Autodesk Fusion 360 part; units mm, degrees
note: some values were not read from the file. Chosen so that the rebuilt part matches the saved one: which bodies a step acts on; which sketch regions a step uses.
(part 3 of 6)
  line L723 (-60.9101, -10.8648) -> (-58.4101, -10.8648)
  line L724 (-6.5, -11.4513) -> (-5.25, -13.6164)
  line L725 (-55.8611, -13.6164) -> (-53.3611, -13.6164)
  line L726 (-68.5324, -10.8648) -> (-67.2824, -8.6997)
  line L727 (-76.1056, -7.9497) -> (-73.6056, -7.9497)
  line L728 (-92.5268, -8.6997) -> (-91.2768, -10.8648)
  line L729 (-72.2824, -8.6997) -> (-71.0324, -10.8648)
  line L730 (-10.299, -12.2013) -> (-11.549, -14.3664)
  line L731 (-5.25, -9.2863) -> (-6.5, -11.4513)
  line L732 (-101.399, -6.5347) -> (-102.649, -8.6997)
  line L733 (-65.9833, -3.6196) -> (-67.2333, -5.7847)
  line L734 (-63.4833, -7.9497) -> (-62.2333, -5.7847)
  line L735 (-71.0324, -10.8648) -> (-68.5324, -10.8648)
  line L736 (-81.1546, -6.5347) -> (-82.4046, -8.6997)
  line L737 (-7.799, -12.2013) -> (-10.299, -12.2013)
  line L738 (-58.4101, -6.5347) -> (-60.9101, -6.5347)
  line L739 (-83.7278, -3.6196) -> (-86.2278, -3.6196)
  line L740 (-2.75, -9.2863) -> (-5.25, -9.2863)
  line L741 (-77.4046, -8.6997) -> (-78.6546, -6.5347)
  line L742 (-10.299, -16.5315) -> (-7.799, -16.5315)
  line L743 (-11.549, -14.3664) -> (-10.299, -16.5315)
  line L744 (-60.9101, -6.5347) -> (-62.1601, -8.6997)
  line L745 (-86.2278, -3.6196) -> (-87.4778, -5.7847)
  line L746 (-15.3722, -13.6164) -> (-12.8722, -13.6164)
  line L747 (-22.9944, -9.2863) -> (-25.4944, -9.2863)
  line L748 (-26.7935, -14.3664) -> (-28.0435, -12.2013)
  line L749 (-48.2879, -12.2013) -> (-50.7879, -12.2013)
  line L750 (-53.3611, -9.2863) -> (-55.8611, -9.2863)
  line L751 (-15.3722, -9.2863) -> (-16.6222, -11.4513)
  line L752 (-46.9889, -11.4513) -> (-45.7389, -13.6164)
  line L753 (-35.6167, -13.6164) -> (-33.1167, -13.6164)
  line L754 (-31.7935, -14.3664) -> (-30.5435, -16.5315)
  line L755 (-6.549, -14.3664) -> (-7.799, -12.2013)
  line L756 (-17.9213, -12.2013) -> (-20.4213, -12.2013)
  line L757 (-60.9101, -12.2013) -> (-62.1601, -14.3664)
  line L758 (-40.6657, -12.2013) -> (-41.9157, -14.3664)
  line L759 (-53.3611, -13.6164) -> (-52.1111, -11.4513)
  line L760 (-26.7444, -11.4513) -> (-25.4944, -13.6164)
  line L761 (-41.9157, -14.3664) -> (-40.6657, -16.5315)
  line L762 (-50.7879, -16.5315) -> (-48.2879, -16.5315)
  line L763 (-60.9101, -16.5315) -> (-58.4101, -16.5315)
  line L764 (-58.4101, -12.2013) -> (-60.9101, -12.2013)
  line L765 (-67.2333, -11.4513) -> (-65.9833, -13.6164)
  line L766 (-28.0435, -16.5315) -> (-26.7935, -14.3664)
  line L767 (-17.9213, -16.5315) -> (-16.6713, -14.3664)
  line L768 (-47.0379, -14.3664) -> (-48.2879, -12.2013)
  line L769 (-12.8722, -13.6164) -> (-11.6222, -11.4513)
  line L770 (-35.6167, -9.2863) -> (-36.8667, -11.4513)
  line L771 (-43.2389, -9.2863) -> (-45.7389, -9.2863)
  line L772 (-57.1111, -11.4513) -> (-55.8611, -13.6164)
  line L773 (-33.1167, -9.2863) -> (-35.6167, -9.2863)
  line L774 (-48.2879, -16.5315) -> (-47.0379, -14.3664)
  line L775 (-30.5435, -16.5315) -> (-28.0435, -16.5315)
  line L776 (-45.7389, -13.6164) -> (-43.2389, -13.6164)
  line L777 (-58.4101, -16.5315) -> (-57.1601, -14.3664)
  line L778 (-30.5435, -12.2013) -> (-31.7935, -14.3664)
  line L779 (-52.0379, -14.3664) -> (-50.7879, -16.5315)
  line L780 (-45.7389, -9.2863) -> (-46.9889, -11.4513)
  line L781 (-55.8611, -9.2863) -> (-57.1111, -11.4513)
  line L782 (-36.9157, -14.3664) -> (-38.1657, -12.2013)
  line L783 (-50.7879, -12.2013) -> (-52.0379, -14.3664)
  line L784 (-43.2389, -13.6164) -> (-41.9889, -11.4513)
  line L785 (-36.8667, -11.4513) -> (-35.6167, -13.6164)
  line L786 (-22.9944, -13.6164) -> (-21.7444, -11.4513)
  line L787 (-20.4213, -16.5315) -> (-17.9213, -16.5315)
  line L788 (-21.6713, -14.3664) -> (-20.4213, -16.5315)
  line L789 (-52.1111, -11.4513) -> (-53.3611, -9.2863)
  line L790 (-28.0435, -12.2013) -> (-30.5435, -12.2013)
  line L791 (-20.4213, -12.2013) -> (-21.6713, -14.3664)
  line L792 (-25.4944, -9.2863) -> (-26.7444, -11.4513)
  line L793 (-7.799, -16.5315) -> (-6.549, -14.3664)
  line L794 (-57.1601, -14.3664) -> (-58.4101, -12.2013)
  line L795 (-12.8722, -9.2863) -> (-15.3722, -9.2863)
  line L796 (-65.9833, -13.6164) -> (-63.4833, -13.6164)
  line L797 (-25.4944, -13.6164) -> (-22.9944, -13.6164)
  line L798 (-40.6657, -16.5315) -> (-38.1657, -16.5315)
  line L799 (-31.8667, -11.4513) -> (-33.1167, -9.2863)
  line L800 (-41.9889, -11.4513) -> (-43.2389, -9.2863)
  line L801 (-38.1657, -12.2013) -> (-40.6657, -12.2013)
  line L802 (-62.1601, -14.3664) -> (-60.9101, -16.5315)
  line L803 (-11.6222, -11.4513) -> (-12.8722, -9.2863)
  line L804 (-21.7444, -11.4513) -> (-22.9944, -9.2863)
  line L805 (-16.6222, -11.4513) -> (-15.3722, -13.6164)
  line L806 (-68.5324, -16.5315) -> (-67.2824, -14.3664)
  line L807 (-38.1657, -16.5315) -> (-36.9157, -14.3664)
  line L808 (-67.2824, -14.3664) -> (-68.5324, -12.2013)
  line L809 (-62.1601, -76.6997) -> (-60.9101, -78.8648)
  line L810 (-86.2278, -71.6196) -> (-87.4778, -73.7847)
  line L811 (-97.6, -73.7847) -> (-96.35, -75.9497)
  line L812 (-87.4778, -73.7847) -> (-86.2278, -75.9497)
  line L813 (-76.1056, -75.9497) -> (-73.6056, -75.9497)
  line L814 (-78.6546, -78.8648) -> (-77.4046, -76.6997)
  line L815 (-77.4046, -76.6997) -> (-78.6546, -74.5347)
  line L816 (-71.0324, -78.8648) -> (-68.5324, -78.8648)
  line L817 (-63.4833, -13.6164) -> (-62.2333, -11.4513)
  line L818 (-33.1167, -13.6164) -> (-31.8667, -11.4513)
  line L819 (-63.4833, -9.2863) -> (-65.9833, -9.2863)
  line L820 (-72.2824, -14.3664) -> (-71.0324, -16.5315)
  line L821 (-71.0324, -12.2013) -> (-72.2824, -14.3664)
  line L822 (-16.6713, -14.3664) -> (-17.9213, -12.2013)
  line L823 (-71.0324, -16.5315) -> (-68.5324, -16.5315)
  line L824 (-60.9101, -78.8648) -> (-58.4101, -78.8648)
  line L825 (-83.7278, -71.6196) -> (-86.2278, -71.6196)
  line L826 (-92.6, -73.7847) -> (-93.85, -71.6196)
  line L827 (-62.2333, -11.4513) -> (-63.4833, -9.2863)
  line L828 (-68.5324, -74.5347) -> (-71.0324, -74.5347)
  line L829 (-65.9833, -9.2863) -> (-67.2333, -11.4513)
  line L830 (-12.8722, -81.6164) -> (-11.6222, -79.4513)
  line L831 (-68.5324, -12.2013) -> (-71.0324, -12.2013)
  line L832 (-16.6222, -79.4513) -> (-15.3722, -81.6164)
  line L833 (-55.8611, -71.6196) -> (-57.1111, -73.7847)
  line L834 (-83.7278, -75.9497) -> (-82.4778, -73.7847)
  line L835 (-91.2768, -78.8648) -> (-88.7768, -78.8648)
  line L836 (-65.9833, -75.9497) -> (-63.4833, -75.9497)
  line L837 (-78.6546, -74.5347) -> (-81.1546, -74.5347)
  line L838 (-58.4101, -74.5347) -> (-60.9101, -74.5347)
  line L839 (-76.1056, -71.6196) -> (-77.3556, -73.7847)
  line L840 (-67.2333, -73.7847) -> (-65.9833, -75.9497)
  line L841 (-92.5268, -76.6997) -> (-91.2768, -78.8648)
  line L842 (-101.399, -78.8648) -> (-98.899, -78.8648)
  line L843 (-97.649, -76.6997) -> (-98.899, -74.5347)
  line L844 (-65.9833, -71.6196) -> (-67.2333, -73.7847)
  line L845 (-68.5324, -78.8648) -> (-67.2824, -76.6997)
  line L846 (-81.1546, -78.8648) -> (-78.6546, -78.8648)
  line L847 (-15.3722, -77.2863) -> (-16.6222, -79.4513)
  line L848 (-96.35, -71.6196) -> (-97.6, -73.7847)
  line L849 (-88.7768, -74.5347) -> (-91.2768, -74.5347)
  line L850 (-72.2824, -76.6997) -> (-71.0324, -78.8648)
  line L851 (-53.3611, -75.9497) -> (-52.1111, -73.7847)
  line L852 (-93.85, -71.6196) -> (-96.35, -71.6196)
  line L853 (-62.2333, -73.7847) -> (-63.4833, -71.6196)
  line L854 (-60.9101, -74.5347) -> (-62.1601, -76.6997)
  line L855 (-77.3556, -73.7847) -> (-76.1056, -75.9497)
  line L856 (-12.8722, -77.2863) -> (-15.3722, -77.2863)
  line L857 (-73.6056, -71.6196) -> (-76.1056, -71.6196)
  line L858 (-88.7768, -78.8648) -> (-87.5268, -76.6997)
  line L859 (-102.649, -76.6997) -> (-101.399, -78.8648)
  line L860 (-82.4778, -73.7847) -> (-83.7278, -71.6196)
  line L861 (-11.6222, -79.4513) -> (-12.8722, -77.2863)
  line L862 (-53.3611, -71.6196) -> (-55.8611, -71.6196)
  line L863 (-52.1111, -73.7847) -> (-53.3611, -71.6196)
  line L864 (-72.3556, -73.7847) -> (-73.6056, -71.6196)
  line L865 (-71.0324, -74.5347) -> (-72.2824, -76.6997)
  line L866 (-67.2824, -76.6997) -> (-68.5324, -74.5347)
  line L867 (-87.5268, -76.6997) -> (-88.7768, -74.5347)
  line L868 (-81.1546, -74.5347) -> (-82.4046, -76.6997)
  line L869 (-58.4101, -78.8648) -> (-57.1601, -76.6997)
  line L870 (-96.35, -75.9497) -> (-93.85, -75.9497)
  line L871 (-101.399, -74.5347) -> (-102.649, -76.6997)
  line L872 (-98.899, -78.8648) -> (-97.649, -76.6997)
  line L873 (-73.6056, -75.9497) -> (-72.3556, -73.7847)
  line L874 (-63.4833, -75.9497) -> (-62.2333, -73.7847)
  line L875 (-82.4046, -76.6997) -> (-81.1546, -78.8648)
  line L876 (-86.2278, -75.9497) -> (-83.7278, -75.9497)
  line L877 (-93.85, -75.9497) -> (-92.6, -73.7847)
  line L878 (-15.3722, -81.6164) -> (-12.8722, -81.6164)
  line L879 (-63.4833, -71.6196) -> (-65.9833, -71.6196)
  line L880 (-57.1601, -76.6997) -> (-58.4101, -74.5347)
  line L881 (-30.5435, -80.2013) -> (-31.7935, -82.3664)
  line L882 (-50.7879, -84.5315) -> (-48.2879, -84.5315)
  line L883 (-53.3611, -81.6164) -> (-52.1111, -79.4513)
  line L884 (-20.4213, -80.2013) -> (-21.6713, -82.3664)
  line L885 (-31.7935, -82.3664) -> (-30.5435, -84.5315)
  line L886 (-58.4101, -84.5315) -> (-57.1601, -82.3664)
  line L887 (-98.899, -74.5347) -> (-101.399, -74.5347)
  line L888 (-25.4944, -81.6164) -> (-22.9944, -81.6164)
  line L889 (-67.2333, -79.4513) -> (-65.9833, -81.6164)
  line L890 (-55.8611, -77.2863) -> (-57.1111, -79.4513)
  line L891 (-58.4101, -80.2013) -> (-60.9101, -80.2013)
  line L892 (-65.9833, -77.2863) -> (-67.2333, -79.4513)
  line L893 (-71.0324, -80.2013) -> (-72.2824, -82.3664)
  line L894 (-63.4833, -77.2863) -> (-65.9833, -77.2863)
  line L895 (-72.2824, -82.3664) -> (-71.0324, -84.5315)
  line L896 (-26.7935, -82.3664) -> (-28.0435, -80.2013)
  line L897 (-57.1111, -79.4513) -> (-55.8611, -81.6164)
  line L898 (-33.1167, -77.2863) -> (-35.6167, -77.2863)
  line L899 (-20.4213, -84.5315) -> (-17.9213, -84.5315)
  line L900 (-45.7389, -81.6164) -> (-43.2389, -81.6164)
  line L901 (-40.6657, -80.2013) -> (-41.9157, -82.3664)
  line L902 (-36.8667, -79.4513) -> (-35.6167, -81.6164)
  line L903 (-91.2768, -74.5347) -> (-92.5268, -76.6997)
  line L904 (-16.6713, -82.3664) -> (-17.9213, -80.2013)
  line L905 (-62.2333, -79.4513) -> (-63.4833, -77.2863)
  line L906 (-48.2879, -80.2013) -> (-50.7879, -80.2013)
  line L907 (-31.8667, -79.4513) -> (-33.1167, -77.2863)
  line L908 (-57.1601, -82.3664) -> (-58.4101, -80.2013)
  line L909 (-65.9833, -81.6164) -> (-63.4833, -81.6164)
  line L910 (-22.9944, -77.2863) -> (-25.4944, -77.2863)
  line L911 (-35.6167, -81.6164) -> (-33.1167, -81.6164)
  line L912 (-40.6657, -84.5315) -> (-38.1657, -84.5315)
  line L913 (-48.2879, -84.5315) -> (-47.0379, -82.3664)
  line L914 (-28.0435, -84.5315) -> (-26.7935, -82.3664)
  line L915 (-71.0324, -84.5315) -> (-68.5324, -84.5315)
  line L916 (-63.4833, -81.6164) -> (-62.2333, -79.4513)
  line L917 (-68.5324, -80.2013) -> (-71.0324, -80.2013)
  line L918 (-30.5435, -84.5315) -> (-28.0435, -84.5315)
  line L919 (-36.9157, -82.3664) -> (-38.1657, -80.2013)
  line L920 (-22.9944, -81.6164) -> (-21.7444, -79.4513)
  line L921 (-41.9889, -79.4513) -> (-43.2389, -77.2863)
  line L922 (-43.2389, -77.2863) -> (-45.7389, -77.2863)
  line L923 (-46.9889, -79.4513) -> (-45.7389, -81.6164)
  line L924 (-28.0435, -80.2013) -> (-30.5435, -80.2013)
  line L925 (-21.7444, -79.4513) -> (-22.9944, -77.2863)
  line L926 (-52.0379, -82.3664) -> (-50.7879, -84.5315)
  line L927 (-47.0379, -82.3664) -> (-48.2879, -80.2013)
  line L928 (-17.9213, -80.2013) -> (-20.4213, -80.2013)
  line L929 (-53.3611, -77.2863) -> (-55.8611, -77.2863)
  line L930 (-17.9213, -84.5315) -> (-16.6713, -82.3664)
  line L931 (-41.9157, -82.3664) -> (-40.6657, -84.5315)
  line L932 (-45.7389, -77.2863) -> (-46.9889, -79.4513)
  line L933 (-21.6713, -82.3664) -> (-20.4213, -84.5315)
  line L934 (-43.2389, -81.6164) -> (-41.9889, -79.4513)
  line L935 (-86.2278, -77.2863) -> (-87.4778, -79.4513)
  line L936 (-55.8611, -81.6164) -> (-53.3611, -81.6164)
  line L937 (-2.75, -87.2831) -> (-1.5, -85.118)
  line L938 (-88.7768, -84.5315) -> (-87.5268, -82.3664)
  line L939 (-73.6056, -81.6164) -> (-72.3556, -79.4513)
  line L940 (-92.5268, -82.3664) -> (-91.2768, -84.5315)
  line L941 (-82.4046, -82.3664) -> (-81.1546, -84.5315)
  line L942 (-96.35, -81.6164) -> (-93.85, -81.6164)
  line L943 (-33.1167, -81.6164) -> (-31.8667, -79.4513)
  line L944 (-38.1657, -80.2013) -> (-40.6657, -80.2013)
  line L945 (-38.1657, -84.5315) -> (-36.9157, -82.3664)
  line L946 (-82.4778, -79.4513) -> (-83.7278, -77.2863)
  line L947 (-93.85, -81.6164) -> (-92.6, -79.4513)
  line L948 (-83.7278, -81.6164) -> (-82.4778, -79.4513)
  line L949 (-25.4944, -77.2863) -> (-26.7444, -79.4513)
  line L950 (-93.85, -77.2863) -> (-96.35, -77.2863)
  line L951 (-62.1601, -82.3664) -> (-60.9101, -84.5315)
  line L952 (-35.6167, -77.2863) -> (-36.8667, -79.4513)
  line L953 (-60.9101, -84.5315) -> (-58.4101, -84.5315)
  line L954 (-60.9101, -80.2013) -> (-62.1601, -82.3664)
  line L955 (-52.1111, -79.4513) -> (-53.3611, -77.2863)
  line L956 (-50.7879, -80.2013) -> (-52.0379, -82.3664)
  line L957 (-26.7444, -79.4513) -> (-25.4944, -81.6164)
  line L958 (-101.399, -84.5315) -> (-98.899, -84.5315)
  line L959 (-7.799, -90.1981) -> (-6.549, -88.0331)
  line L960 (-91.2768, -80.2013) -> (-92.5268, -82.3664)
  line L961 (-72.3556, -79.4513) -> (-73.6056, -77.2863)
  line L962 (-102.649, -82.3664) -> (-101.399, -84.5315)
  line L963 (-101.399, -80.2013) -> (-102.649, -82.3664)
  line L964 (-21.6713, -88.0331) -> (-20.4213, -90.1981)
  line L965 (-76.1056, -77.2863) -> (-77.3556, -79.4513)
  line L966 (-16.6222, -85.118) -> (-15.3722, -87.2831)
  line L967 (-15.3722, -82.9529) -> (-16.6222, -85.118)
  line L968 (-20.4213, -90.1981) -> (-17.9213, -90.1981)
  line L969 (-11.6222, -85.118) -> (-12.8722, -82.9529)
  line L970 (-2.75, -82.9529) -> (-5.25, -82.9529)
  line L971 (-5.25, -82.9529) -> (-6.5, -85.118)
  line L972 (-92.6, -79.4513) -> (-93.85, -77.2863)
  line L973 (-78.6546, -80.2013) -> (-81.1546, -80.2013)
  line L974 (-83.7278, -77.2863) -> (-86.2278, -77.2863)
  line L975 (-88.7768, -80.2013) -> (-91.2768, -80.2013)
  line L976 (-7.799, -85.868) -> (-10.299, -85.868)
  line L977 (-98.899, -80.2013) -> (-101.399, -80.2013)
  line L978 (-81.1546, -80.2013) -> (-82.4046, -82.3664)
  line L979 (-87.5268, -82.3664) -> (-88.7768, -80.2013)
  line L980 (-12.8722, -87.2831) -> (-11.6222, -85.118)
  line L981 (-17.9213, -85.868) -> (-20.4213, -85.868)
  line L982 (-20.4213, -85.868) -> (-21.6713, -88.0331)
  line L983 (-67.2824, -82.3664) -> (-68.5324, -80.2013)
  line L984 (-96.35, -77.2863) -> (-97.6, -79.4513)
  line L985 (-10.299, -85.868) -> (-11.549, -88.0331)
  line L986 (-1.5, -85.118) -> (-2.75, -82.9529)
  line L987 (-17.9213, -90.1981) -> (-16.6713, -88.0331)
  line L988 (-16.6713, -88.0331) -> (-17.9213, -85.868)
  line L989 (-98.899, -84.5315) -> (-97.649, -82.3664)
  line L990 (-6.5, -85.118) -> (-5.25, -87.2831)
  line L991 (-77.4046, -82.3664) -> (-78.6546, -80.2013)
  line L992 (-5.25, -87.2831) -> (-2.75, -87.2831)
  line L993 (-6.549, -88.0331) -> (-7.799, -85.868)
  line L994 (-25.4944, -87.2831) -> (-22.9944, -87.2831)
  line L995 (-73.6056, -77.2863) -> (-76.1056, -77.2863)
  line L996 (-12.8722, -82.9529) -> (-15.3722, -82.9529)
  line L997 (-81.1546, -84.5315) -> (-78.6546, -84.5315)
  line L998 (-10.299, -90.1981) -> (-7.799, -90.1981)
  line L999 (-15.3722, -87.2831) -> (-12.8722, -87.2831)
  line L1000 (-11.549, -88.0331) -> (-10.299, -90.1981)
  line L1001 (-97.6, -79.4513) -> (-96.35, -81.6164)
  line L1002 (-97.649, -82.3664) -> (-98.899, -80.2013)
  line L1003 (-87.4778, -79.4513) -> (-86.2278, -81.6164)
  line L1004 (-86.2278, -81.6164) -> (-83.7278, -81.6164)
  line L1005 (-77.3556, -79.4513) -> (-76.1056, -81.6164)
  line L1006 (-91.2768, -84.5315) -> (-88.7768, -84.5315)
  line L1007 (-26.7444, -85.118) -> (-25.4944, -87.2831)
  line L1008 (-25.4944, -111.2863) -> (-26.7444, -113.4513)
  line L1009 (-40.6657, -118.5315) -> (-38.1657, -118.5315)
  line L1010 (-33.1167, -111.2863) -> (-35.6167, -111.2863)
  line L1011 (-53.3611, -111.2863) -> (-55.8611, -111.2863)
  line L1012 (-53.3611, -115.6164) -> (-52.1111, -113.4513)
  line L1013 (-52.1111, -113.4513) -> (-53.3611, -111.2863)
  line L1014 (-22.9944, -111.2863) -> (-25.4944, -111.2863)
  line L1015 (-21.7444, -113.4513) -> (-22.9944, -111.2863)
  line L1016 (-10.299, -118.5315) -> (-7.799, -118.5315)
  line L1017 (-7.799, -114.2013) -> (-10.299, -114.2013)
  line L1018 (-36.8667, -113.4513) -> (-35.6167, -115.6164)
  line L1019 (-31.8667, -113.4513) -> (-33.1167, -111.2863)
  line L1020 (-33.1167, -115.6164) -> (-31.8667, -113.4513)
  line L1021 (-48.2879, -114.2013) -> (-50.7879, -114.2013)
  line L1022 (-50.7879, -118.5315) -> (-48.2879, -118.5315)
  line L1023 (-55.8611, -111.2863) -> (-57.1111, -113.4513)
  line L1024 (-50.7879, -114.2013) -> (-52.0379, -116.3664)
  line L1025 (-15.3722, -115.6164) -> (-12.8722, -115.6164)
  line L1026 (-28.0435, -114.2013) -> (-30.5435, -114.2013)
  line L1027 (-26.7935, -116.3664) -> (-28.0435, -114.2013)
  line L1028 (-36.9157, -116.3664) -> (-38.1657, -114.2013)
  line L1029 (-11.549, -116.3664) -> (-10.299, -118.5315)
  line L1030 (-38.1657, -114.2013) -> (-40.6657, -114.2013)
  line L1031 (-47.0379, -116.3664) -> (-48.2879, -114.2013)
  line L1032 (-52.0379, -116.3664) -> (-50.7879, -118.5315)
  line L1033 (-17.9213, -118.5315) -> (-16.6713, -116.3664)
  line L1034 (-6.549, -116.3664) -> (-7.799, -114.2013)
  line L1035 (-15.3722, -111.2863) -> (-16.6222, -113.4513)
  line L1036 (-1.5, -113.4513) -> (-2.75, -111.2863)
  line L1037 (-40.6657, -114.2013) -> (-41.9157, -116.3664)
  line L1038 (-12.8722, -115.6164) -> (-11.6222, -113.4513)
  line L1039 (-5.25, -111.2863) -> (-6.5, -113.4513)
  line L1040 (-45.7389, -115.6164) -> (-43.2389, -115.6164)
  line L1041 (-21.6713, -116.3664) -> (-20.4213, -118.5315)
  line L1042 (-25.4944, -115.6164) -> (-22.9944, -115.6164)
  line L1043 (-2.75, -115.6164) -> (-1.5, -113.4513)
  line L1044 (-41.9157, -116.3664) -> (-40.6657, -118.5315)
  line L1045 (-35.6167, -115.6164) -> (-33.1167, -115.6164)
  line L1046 (-16.6713, -116.3664) -> (-17.9213, -114.2013)
  line L1047 (-43.2389, -111.2863) -> (-45.7389, -111.2863)
  line L1048 (-16.6222, -113.4513) -> (-15.3722, -115.6164)
  line L1049 (-31.7935, -116.3664) -> (-30.5435, -118.5315)
  line L1050 (-93.85, -115.6164) -> (-92.6, -113.4513)
  line L1051 (-98.899, -118.5315) -> (-97.649, -116.3664)
  line L1052 (-7.799, -118.5315) -> (-6.549, -116.3664)
  line L1053 (-6.5, -119.118) -> (-5.25, -121.2831)
  line L1054 (-26.7444, -113.4513) -> (-25.4944, -115.6164)
  line L1055 (-81.1546, -118.5315) -> (-78.6546, -118.5315)
  line L1056 (-30.5435, -118.5315) -> (-28.0435, -118.5315)
  line L1057 (-92.6, -113.4513) -> (-93.85, -111.2863)
  line L1058 (-96.35, -111.2863) -> (-97.6, -113.4513)
  line L1059 (-78.6546, -114.2013) -> (-81.1546, -114.2013)
  line L1060 (-68.5324, -118.5315) -> (-67.2824, -116.3664)
  line L1061 (-67.2824, -116.3664) -> (-68.5324, -114.2013)
  line L1062 (-60.9101, -114.2013) -> (-62.1601, -116.3664)
  line L1063 (-63.4833, -111.2863) -> (-65.9833, -111.2863)
  line L1064 (-73.6056, -115.6164) -> (-72.3556, -113.4513)
  line L1065 (-5.25, -121.2831) -> (-2.75, -121.2831)
  line L1066 (-88.7768, -118.5315) -> (-87.5268, -116.3664)
  line L1067 (-2.75, -121.2831) -> (-1.5, -119.118)
  line L1068 (-1.5, -119.118) -> (-2.75, -116.9529)
  line L1069 (-5.25, -116.9529) -> (-6.5, -119.118)
  line L1070 (-86.2278, -111.2863) -> (-87.4778, -113.4513)
  line L1071 (-10.299, -119.868) -> (-11.549, -122.0331)
  line L1072 (-58.4101, -114.2013) -> (-60.9101, -114.2013)
  line L1073 (-83.7278, -111.2863) -> (-86.2278, -111.2863)
  line L1074 (-62.2333, -113.4513) -> (-63.4833, -111.2863)
  line L1075 (-77.4046, -116.3664) -> (-78.6546, -114.2013)
  line L1076 (-92.5268, -116.3664) -> (-91.2768, -118.5315)
  line L1077 (-65.9833, -111.2863) -> (-67.2333, -113.4513)
  line L1078 (-86.2278, -115.6164) -> (-83.7278, -115.6164)
  line L1079 (-72.2824, -116.3664) -> (-71.0324, -118.5315)
  line L1080 (-71.0324, -118.5315) -> (-68.5324, -118.5315)
  line L1081 (-73.6056, -111.2863) -> (-76.1056, -111.2863)
  line L1082 (-77.3556, -113.4513) -> (-76.1056, -115.6164)
  line L1083 (-58.4101, -118.5315) -> (-57.1601, -116.3664)
  line L1084 (-57.1601, -116.3664) -> (-58.4101, -114.2013)
  line L1085 (-91.2768, -118.5315) -> (-88.7768, -118.5315)
  line L1086 (-7.799, -119.868) -> (-10.299, -119.868)
  line L1087 (-72.3556, -113.4513) -> (-73.6056, -111.2863)
  line L1088 (-78.6546, -118.5315) -> (-77.4046, -116.3664)
  line L1089 (-101.399, -118.5315) -> (-98.899, -118.5315)
  line L1090 (-67.2333, -113.4513) -> (-65.9833, -115.6164)
  line L1091 (-11.549, -122.0331) -> (-10.299, -124.1981)
  line L1092 (-101.399, -114.2013) -> (-102.649, -116.3664)
  line L1093 (-87.5268, -116.3664) -> (-88.7768, -114.2013)
  line L1094 (-98.899, -114.2013) -> (-101.399, -114.2013)
  line L1095 (-10.299, -124.1981) -> (-7.799, -124.1981)
  line L1096 (-83.7278, -115.6164) -> (-82.4778, -113.4513)
  line L1097 (-97.649, -116.3664) -> (-98.899, -114.2013)
  line L1098 (-76.1056, -111.2863) -> (-77.3556, -113.4513)
  line L1099 (-63.4833, -115.6164) -> (-62.2333, -113.4513)
  line L1100 (-60.9101, -118.5315) -> (-58.4101, -118.5315)
  line L1101 (-2.75, -116.9529) -> (-5.25, -116.9529)
  line L1102 (-91.2768, -114.2013) -> (-92.5268, -116.3664)
  line L1103 (-71.0324, -114.2013) -> (-72.2824, -116.3664)
  line L1104 (-88.7768, -114.2013) -> (-91.2768, -114.2013)
  line L1105 (-65.9833, -115.6164) -> (-63.4833, -115.6164)
  line L1106 (-82.4046, -116.3664) -> (-81.1546, -118.5315)
  line L1107 (-82.4778, -113.4513) -> (-83.7278, -111.2863)
  line L1108 (-41.9889, -119.118) -> (-43.2389, -116.9529)
  line L1109 (-46.9889, -119.118) -> (-45.7389, -121.2831)
  line L1110 (-96.35, -115.6164) -> (-93.85, -115.6164)
  line L1111 (-41.9157, -122.0331) -> (-40.6657, -124.1981)
  line L1112 (-17.9213, -124.1981) -> (-16.6713, -122.0331)
  line L1113 (-97.6, -113.4513) -> (-96.35, -115.6164)
  line L1114 (-81.1546, -114.2013) -> (-82.4046, -116.3664)
  line L1115 (-87.4778, -113.4513) -> (-86.2278, -115.6164)
  line L1116 (-22.9944, -121.2831) -> (-21.7444, -119.118)
  line L1117 (-93.85, -111.2863) -> (-96.35, -111.2863)
  line L1118 (-12.8722, -116.9529) -> (-15.3722, -116.9529)
  line L1119 (-33.1167, -121.2831) -> (-31.8667, -119.118)
  line L1120 (-62.1601, -116.3664) -> (-60.9101, -118.5315)
  line L1121 (-38.1657, -119.868) -> (-40.6657, -119.868)
  line L1122 (-50.7879, -124.1981) -> (-48.2879, -124.1981)
  line L1123 (-40.6657, -124.1981) -> (-38.1657, -124.1981)
  line L1124 (-68.5324, -114.2013) -> (-71.0324, -114.2013)
  line L1125 (-102.649, -116.3664) -> (-101.399, -118.5315)
  line L1126 (-30.5435, -124.1981) -> (-28.0435, -124.1981)
  line L1127 (-28.0435, -119.868) -> (-30.5435, -119.868)
  line L1128 (-45.7389, -116.9529) -> (-46.9889, -119.118)
  line L1129 (-48.2879, -119.868) -> (-50.7879, -119.868)
  line L1130 (-48.2879, -124.1981) -> (-47.0379, -122.0331)
  line L1131 (-45.7389, -121.2831) -> (-43.2389, -121.2831)
  line L1132 (-76.1056, -115.6164) -> (-73.6056, -115.6164)
  line L1133 (-16.6713, -122.0331) -> (-17.9213, -119.868)
  line L1134 (-21.7444, -119.118) -> (-22.9944, -116.9529)
  line L1135 (-6.549, -122.0331) -> (-7.799, -119.868)
  line L1136 (-38.1657, -124.1981) -> (-36.9157, -122.0331)
  line L1137 (-57.1111, -119.118) -> (-55.8611, -121.2831)
  line L1138 (-33.1167, -116.9529) -> (-35.6167, -116.9529)
  line L1139 (-55.8611, -121.2831) -> (-53.3611, -121.2831)
  line L1140 (-16.6222, -119.118) -> (-15.3722, -121.2831)
  line L1141 (-20.4213, -124.1981) -> (-17.9213, -124.1981)
  line L1142 (-7.799, -124.1981) -> (-6.549, -122.0331)
  line L1143 (-22.9944, -116.9529) -> (-25.4944, -116.9529)
  line L1144 (-43.2389, -121.2831) -> (-41.9889, -119.118)
  line L1145 (-53.3611, -121.2831) -> (-52.1111, -119.118)
  line L1146 (-52.1111, -119.118) -> (-53.3611, -116.9529)
  line L1147 (-55.8611, -116.9529) -> (-57.1111, -119.118)
  line L1148 (-31.8667, -119.118) -> (-33.1167, -116.9529)
  line L1149 (-53.3611, -116.9529) -> (-55.8611, -116.9529)
  line L1150 (-58.4101, -119.868) -> (-60.9101, -119.868)
  line L1151 (-28.0435, -124.1981) -> (-26.7935, -122.0331)
  line L1152 (-26.7935, -122.0331) -> (-28.0435, -119.868)
  line L1153 (-47.0379, -122.0331) -> (-48.2879, -119.868)
  line L1154 (-62.1601, -122.0331) -> (-60.9101, -124.1981)
  line L1155 (-21.6713, -122.0331) -> (-20.4213, -124.1981)
  line L1156 (-26.7444, -119.118) -> (-25.4944, -121.2831)
  line L1157 (-60.9101, -124.1981) -> (-58.4101, -124.1981)
  line L1158 (-46.9889, -113.4513) -> (-45.7389, -115.6164)
  line L1159 (-43.2389, -115.6164) -> (-41.9889, -113.4513)
  line L1160 (-28.0435, -118.5315) -> (-26.7935, -116.3664)
  line L1161 (-78.6546, -112.8648) -> (-77.4046, -110.6997)
  line L1162 (-83.7278, -109.9497) -> (-82.4778, -107.7847)
  line L1163 (-30.5435, -114.2013) -> (-31.7935, -116.3664)
  line L1164 (-35.6167, -111.2863) -> (-36.8667, -113.4513)
  line L1165 (-20.4213, -118.5315) -> (-17.9213, -118.5315)
  line L1166 (-38.1657, -118.5315) -> (-36.9157, -116.3664)
  line L1167 (-41.9889, -113.4513) -> (-43.2389, -111.2863)
  line L1168 (-45.7389, -111.2863) -> (-46.9889, -113.4513)
  line L1169 (-11.6222, -113.4513) -> (-12.8722, -111.2863)
  line L1170 (-2.75, -111.2863) -> (-5.25, -111.2863)
  line L1171 (-48.2879, -118.5315) -> (-47.0379, -116.3664)
  line L1172 (-57.1111, -113.4513) -> (-55.8611, -115.6164)
  line L1173 (-55.8611, -115.6164) -> (-53.3611, -115.6164)
  line L1174 (-81.1546, -112.8648) -> (-78.6546, -112.8648)
  line L1175 (-17.9213, -114.2013) -> (-20.4213, -114.2013)
  line L1176 (-12.8722, -111.2863) -> (-15.3722, -111.2863)
  line L1177 (-22.9944, -115.6164) -> (-21.7444, -113.4513)
  line L1178 (-20.4213, -114.2013) -> (-21.6713, -116.3664)
  line L1179 (-10.299, -114.2013) -> (-11.549, -116.3664)
  line L1180 (-101.399, -119.868) -> (-102.649, -122.0331)
  line L1181 (-73.6056, -116.9529) -> (-76.1056, -116.9529)
  line L1182 (-40.6657, -119.868) -> (-41.9157, -122.0331)
  line L1183 (-82.4778, -119.118) -> (-83.7278, -116.9529)
  line L1184 (-88.7768, -119.868) -> (-91.2768, -119.868)
  line L1185 (-11.6222, -119.118) -> (-12.8722, -116.9529)
  line L1186 (-96.35, -121.2831) -> (-93.85, -121.2831)
  line L1187 (-83.7278, -121.2831) -> (-82.4778, -119.118)
  line L1188 (-1.5, -124.7847) -> (-2.75, -122.6196)
  line L1189 (-91.2768, -124.1981) -> (-88.7768, -124.1981)
  line L1190 (-63.4833, -121.2831) -> (-62.2333, -119.118)
  line L1191 (-52.0379, -122.0331) -> (-50.7879, -124.1981)
  line L1192 (-15.3722, -121.2831) -> (-12.8722, -121.2831)
  line L1193 (-25.4944, -121.2831) -> (-22.9944, -121.2831)
  line L1194 (-91.2768, -119.868) -> (-92.5268, -122.0331)
  line L1195 (-12.8722, -121.2831) -> (-11.6222, -119.118)
  line L1196 (-68.5324, -119.868) -> (-71.0324, -119.868)
  line L1197 (-57.1601, -122.0331) -> (-58.4101, -119.868)
  line L1198 (-50.7879, -119.868) -> (-52.0379, -122.0331)
  line L1199 (-93.85, -116.9529) -> (-96.35, -116.9529)
  line L1200 (-43.2389, -116.9529) -> (-45.7389, -116.9529)
  line L1201 (-36.8667, -119.118) -> (-35.6167, -121.2831)
  line L1202 (-58.4101, -124.1981) -> (-57.1601, -122.0331)
  line L1203 (-78.6546, -119.868) -> (-81.1546, -119.868)
  line L1204 (-25.4944, -116.9529) -> (-26.7444, -119.118)
  line L1205 (-76.1056, -121.2831) -> (-73.6056, -121.2831)
  line L1206 (-92.5268, -122.0331) -> (-91.2768, -124.1981)
  line L1207 (-31.7935, -122.0331) -> (-30.5435, -124.1981)
  line L1208 (-83.7278, -116.9529) -> (-86.2278, -116.9529)
  line L1209 (-6.5, -124.7847) -> (-5.25, -126.9497)
  line L1210 (-98.899, -124.1981) -> (-97.649, -122.0331)
  line L1211 (-11.549, -127.6997) -> (-10.299, -129.8648)
  line L1212 (-97.6, -119.118) -> (-96.35, -121.2831)
  line L1213 (-20.4213, -119.868) -> (-21.6713, -122.0331)
  line L1214 (-98.899, -119.868) -> (-101.399, -119.868)
  line L1215 (-102.649, -122.0331) -> (-101.399, -124.1981)
  line L1216 (-73.6056, -121.2831) -> (-72.3556, -119.118)
  line L1217 (-76.1056, -116.9529) -> (-77.3556, -119.118)
  line L1218 (-96.35, -116.9529) -> (-97.6, -119.118)
  line L1219 (-67.2333, -119.118) -> (-65.9833, -121.2831)
  line L1220 (-86.2278, -121.2831) -> (-83.7278, -121.2831)
  line L1221 (-63.4833, -116.9529) -> (-65.9833, -116.9529)
  line L1222 (-78.6546, -124.1981) -> (-77.4046, -122.0331)
  line L1223 (-101.399, -124.1981) -> (-98.899, -124.1981)
  line L1224 (-7.799, -129.8648) -> (-6.549, -127.6997)
  line L1225 (-35.6167, -116.9529) -> (-36.8667, -119.118)
  line L1226 (-60.9101, -119.868) -> (-62.1601, -122.0331)
  line L1227 (-77.3556, -119.118) -> (-76.1056, -121.2831)
  line L1228 (-17.9213, -119.868) -> (-20.4213, -119.868)
  line L1229 (-97.649, -122.0331) -> (-98.899, -119.868)
  line L1230 (-87.4778, -119.118) -> (-86.2278, -121.2831)
  line L1231 (-62.2333, -119.118) -> (-63.4833, -116.9529)
  line L1232 (-2.75, -122.6196) -> (-5.25, -122.6196)
  line L1233 (-35.6167, -121.2831) -> (-33.1167, -121.2831)
  line L1234 (-86.2278, -116.9529) -> (-87.4778, -119.118)
  line L1235 (-5.25, -122.6196) -> (-6.5, -124.7847)
  line L1236 (-30.5435, -119.868) -> (-31.7935, -122.0331)
  line L1237 (-36.9157, -122.0331) -> (-38.1657, -119.868)
  line L1238 (-88.7768, -124.1981) -> (-87.5268, -122.0331)
  line L1239 (-5.25, -126.9497) -> (-2.75, -126.9497)
  line L1240 (-65.9833, -121.2831) -> (-63.4833, -121.2831)
  line L1241 (-72.3556, -119.118) -> (-73.6056, -116.9529)
  line L1242 (-67.2824, -122.0331) -> (-68.5324, -119.868)
  line L1243 (-15.3722, -116.9529) -> (-16.6222, -119.118)
  line L1244 (-60.9101, -125.5347) -> (-62.1601, -127.6997)
  line L1245 (-15.3722, -126.9497) -> (-12.8722, -126.9497)
  line L1246 (-63.4833, -122.6196) -> (-65.9833, -122.6196)
  line L1247 (-7.799, -125.5347) -> (-10.299, -125.5347)
  line L1248 (-71.0324, -119.868) -> (-72.2824, -122.0331)
  line L1249 (-81.1546, -124.1981) -> (-78.6546, -124.1981)
  line L1250 (-35.6167, -126.9497) -> (-33.1167, -126.9497)
  line L1251 (-12.8722, -126.9497) -> (-11.6222, -124.7847)
  line L1252 (-92.6, -119.118) -> (-93.85, -116.9529)
  line L1253 (-31.7935, -127.6997) -> (-30.5435, -129.8648)
  line L1254 (-68.5324, -124.1981) -> (-67.2824, -122.0331)
  line L1255 (-71.0324, -129.8648) -> (-68.5324, -129.8648)
  line L1256 (-41.9889, -124.7847) -> (-43.2389, -122.6196)
  line L1257 (-20.4213, -125.5347) -> (-21.6713, -127.6997)
  line L1258 (-72.2824, -122.0331) -> (-71.0324, -124.1981)
  line L1259 (-15.3722, -122.6196) -> (-16.6222, -124.7847)
  line L1260 (-87.5268, -122.0331) -> (-88.7768, -119.868)
  line L1261 (-93.85, -121.2831) -> (-92.6, -119.118)
  line L1262 (-10.299, -125.5347) -> (-11.549, -127.6997)
  line L1263 (-53.3611, -122.6196) -> (-55.8611, -122.6196)
  line L1264 (-65.9833, -126.9497) -> (-63.4833, -126.9497)
  line L1265 (-65.9833, -116.9529) -> (-67.2333, -119.118)
  line L1266 (-25.4944, -126.9497) -> (-22.9944, -126.9497)
  line L1267 (-10.299, -129.8648) -> (-7.799, -129.8648)
  line L1268 (-45.7389, -122.6196) -> (-46.9889, -124.7847)
  line L1269 (-72.2824, -127.6997) -> (-71.0324, -129.8648)
  line L1270 (-12.8722, -122.6196) -> (-15.3722, -122.6196)
  line L1271 (-50.7879, -125.5347) -> (-52.0379, -127.6997)
  line L1272 (-47.0379, -127.6997) -> (-48.2879, -125.5347)
  line L1273 (-38.1657, -125.5347) -> (-40.6657, -125.5347)
  line L1274 (-33.1167, -122.6196) -> (-35.6167, -122.6196)
  line L1275 (-36.9157, -127.6997) -> (-38.1657, -125.5347)
  line L1276 (-30.5435, -129.8648) -> (-28.0435, -129.8648)
  line L1277 (-40.6657, -125.5347) -> (-41.9157, -127.6997)
  line L1278 (-52.0379, -127.6997) -> (-50.7879, -129.8648)
  line L1279 (-31.8667, -124.7847) -> (-33.1167, -122.6196)
  line L1280 (-71.0324, -124.1981) -> (-68.5324, -124.1981)
  line L1281 (-45.7389, -126.9497) -> (-43.2389, -126.9497)
  line L1282 (-17.9213, -129.8648) -> (-16.6713, -127.6997)
  line L1283 (-46.9889, -124.7847) -> (-45.7389, -126.9497)
  line L1284 (-43.2389, -126.9497) -> (-41.9889, -124.7847)
  line L1285 (-82.4046, -122.0331) -> (-81.1546, -124.1981)
  line L1286 (-6.549, -127.6997) -> (-7.799, -125.5347)
  line L1287 (-71.0324, -125.5347) -> (-72.2824, -127.6997)
  line L1288 (-50.7879, -129.8648) -> (-48.2879, -129.8648)
  line L1289 (-48.2879, -125.5347) -> (-50.7879, -125.5347)
  line L1290 (-60.9101, -129.8648) -> (-58.4101, -129.8648)
  line L1291 (-55.8611, -126.9497) -> (-53.3611, -126.9497)
  line L1292 (-28.0435, -129.8648) -> (-26.7935, -127.6997)
  line L1293 (-2.75, -126.9497) -> (-1.5, -124.7847)
  line L1294 (-11.6222, -124.7847) -> (-12.8722, -122.6196)
  line L1295 (-81.1546, -119.868) -> (-82.4046, -122.0331)
  line L1296 (-25.4944, -122.6196) -> (-26.7444, -124.7847)
  line L1297 (-38.1657, -129.8648) -> (-36.9157, -127.6997)
  line L1298 (-30.5435, -125.5347) -> (-31.7935, -127.6997)
  line L1299 (-16.6222, -124.7847) -> (-15.3722, -126.9497)
  line L1300 (-20.4213, -129.8648) -> (-17.9213, -129.8648)
  line L1301 (-53.3611, -126.9497) -> (-52.1111, -124.7847)
  line L1302 (-21.6713, -127.6997) -> (-20.4213, -129.8648)
  line L1303 (-26.7935, -127.6997) -> (-28.0435, -125.5347)
  line L1304 (-16.6713, -127.6997) -> (-17.9213, -125.5347)
  line L1305 (-55.8611, -122.6196) -> (-57.1111, -124.7847)
  line L1306 (-57.1601, -127.6997) -> (-58.4101, -125.5347)
  line L1307 (-77.4046, -122.0331) -> (-78.6546, -119.868)
  line L1308 (-83.7278, -122.6196) -> (-86.2278, -122.6196)
  line L1309 (-7.799, -135.5315) -> (-6.549, -133.3664)
  line L1310 (-72.3556, -124.7847) -> (-73.6056, -122.6196)
  line L1311 (-88.7768, -125.5347) -> (-91.2768, -125.5347)
  line L1312 (-63.4833, -126.9497) -> (-62.2333, -124.7847)
  line L1313 (-17.9213, -131.2013) -> (-20.4213, -131.2013)
  line L1314 (-86.2278, -126.9497) -> (-83.7278, -126.9497)
  line L1315 (-22.9944, -126.9497) -> (-21.7444, -124.7847)
  line L1316 (-57.1111, -124.7847) -> (-55.8611, -126.9497)
  line L1317 (-2.75, -132.6164) -> (-1.5, -130.4513)
  line L1318 (-15.3722, -132.6164) -> (-12.8722, -132.6164)
  line L1319 (-11.549, -133.3664) -> (-10.299, -135.5315)
  line L1320 (-91.2768, -129.8648) -> (-88.7768, -129.8648)
  line L1321 (-62.2333, -124.7847) -> (-63.4833, -122.6196)
  line L1322 (-77.4046, -127.6997) -> (-78.6546, -125.5347)
  line L1323 (-81.1546, -125.5347) -> (-82.4046, -127.6997)
  line L1324 (-62.1601, -127.6997) -> (-60.9101, -129.8648)
  line L1325 (-101.399, -129.8648) -> (-98.899, -129.8648)
  line L1326 (-12.8722, -128.2863) -> (-15.3722, -128.2863)
  line L1327 (-92.5268, -127.6997) -> (-91.2768, -129.8648)
  line L1328 (-2.75, -128.2863) -> (-5.25, -128.2863)
  line L1329 (-11.6222, -130.4513) -> (-12.8722, -128.2863)
  line L1330 (-12.8722, -132.6164) -> (-11.6222, -130.4513)
  line L1331 (-26.7444, -124.7847) -> (-25.4944, -126.9497)
  line L1332 (-58.4101, -125.5347) -> (-60.9101, -125.5347)
  line L1333 (-88.7768, -129.8648) -> (-87.5268, -127.6997)
  line L1334 (-91.2768, -125.5347) -> (-92.5268, -127.6997)
  line L1335 (-97.649, -127.6997) -> (-98.899, -125.5347)
  line L1336 (-21.7444, -124.7847) -> (-22.9944, -122.6196)
  line L1337 (-43.2389, -122.6196) -> (-45.7389, -122.6196)
  line L1338 (-67.2824, -127.6997) -> (-68.5324, -125.5347)
  line L1339 (-10.299, -131.2013) -> (-11.549, -133.3664)
  line L1340 (-68.5324, -129.8648) -> (-67.2824, -127.6997)
  line L1341 (-96.35, -126.9497) -> (-93.85, -126.9497)
  line L1342 (-40.6657, -129.8648) -> (-38.1657, -129.8648)
  line L1343 (-15.3722, -128.2863) -> (-16.6222, -130.4513)
  line L1344 (-92.6, -124.7847) -> (-93.85, -122.6196)
  line L1345 (-26.7444, -130.4513) -> (-25.4944, -132.6164)
  line L1346 (-33.1167, -126.9497) -> (-31.8667, -124.7847)
  line L1347 (-68.5324, -125.5347) -> (-71.0324, -125.5347)
  line L1348 (-17.9213, -125.5347) -> (-20.4213, -125.5347)
  line L1349 (-48.2879, -129.8648) -> (-47.0379, -127.6997)
  line L1350 (-97.6, -124.7847) -> (-96.35, -126.9497)
  line L1351 (-35.6167, -122.6196) -> (-36.8667, -124.7847)
  line L1352 (-58.4101, -129.8648) -> (-57.1601, -127.6997)
  line L1353 (-67.2333, -124.7847) -> (-65.9833, -126.9497)
  line L1354 (-102.649, -127.6997) -> (-101.399, -129.8648)
  line L1355 (-10.299, -135.5315) -> (-7.799, -135.5315)
  line L1356 (-17.9213, -135.5315) -> (-16.6713, -133.3664)
  line L1357 (-22.9944, -122.6196) -> (-25.4944, -122.6196)
  line L1358 (-6.549, -133.3664) -> (-7.799, -131.2013)
  line L1359 (-36.8667, -124.7847) -> (-35.6167, -126.9497)
  line L1360 (-28.0435, -125.5347) -> (-30.5435, -125.5347)
  line L1361 (-65.9833, -122.6196) -> (-67.2333, -124.7847)
  line L1362 (-20.4213, -131.2013) -> (-21.6713, -133.3664)
  line L1363 (-93.85, -126.9497) -> (-92.6, -124.7847)
  line L1364 (-78.6546, -129.8648) -> (-77.4046, -127.6997)
  line L1365 (-6.5, -130.4513) -> (-5.25, -132.6164)
  line L1366 (-21.6713, -133.3664) -> (-20.4213, -135.5315)
  line L1367 (-41.9157, -127.6997) -> (-40.6657, -129.8648)
  line L1368 (-7.799, -131.2013) -> (-10.299, -131.2013)
  line L1369 (-87.4778, -124.7847) -> (-86.2278, -126.9497)
  line L1370 (-93.85, -122.6196) -> (-96.35, -122.6196)
  line L1371 (-52.1111, -124.7847) -> (-53.3611, -122.6196)
  line L1372 (-98.899, -129.8648) -> (-97.649, -127.6997)
  line L1373 (-1.5, -130.4513) -> (-2.75, -128.2863)
  line L1374 (-76.1056, -122.6196) -> (-77.3556, -124.7847)
  line L1375 (-73.6056, -132.6164) -> (-72.3556, -130.4513)
  line L1376 (-36.9157, -133.3664) -> (-38.1657, -131.2013)
  line L1377 (-82.4778, -124.7847) -> (-83.7278, -122.6196)
  line L1378 (-55.8611, -132.6164) -> (-53.3611, -132.6164)
  line L1379 (-22.9944, -132.6164) -> (-21.7444, -130.4513)
  line L1380 (-30.5435, -131.2013) -> (-31.7935, -133.3664)
  line L1381 (-62.2333, -130.4513) -> (-63.4833, -128.2863)
  line L1382 (-20.4213, -135.5315) -> (-17.9213, -135.5315)
  line L1383 (-82.4046, -127.6997) -> (-81.1546, -129.8648)
  line L1384 (-76.1056, -126.9497) -> (-73.6056, -126.9497)
  line L1385 (-67.2824, -133.3664) -> (-68.5324, -131.2013)
  line L1386 (-26.7935, -133.3664) -> (-28.0435, -131.2013)
  line L1387 (-87.5268, -127.6997) -> (-88.7768, -125.5347)
  line L1388 (-50.7879, -131.2013) -> (-52.0379, -133.3664)
  line L1389 (-16.6222, -130.4513) -> (-15.3722, -132.6164)
  line L1390 (-63.4833, -128.2863) -> (-65.9833, -128.2863)
  line L1391 (-45.7389, -132.6164) -> (-43.2389, -132.6164)
  line L1392 (-50.7879, -135.5315) -> (-48.2879, -135.5315)
  line L1393 (-48.2879, -135.5315) -> (-47.0379, -133.3664)
  line L1394 (-16.6713, -133.3664) -> (-17.9213, -131.2013)
  line L1395 (-86.2278, -122.6196) -> (-87.4778, -124.7847)
  line L1396 (-101.399, -125.5347) -> (-102.649, -127.6997)
  line L1397 (-73.6056, -122.6196) -> (-76.1056, -122.6196)
  line L1398 (-38.1657, -135.5315) -> (-36.9157, -133.3664)
  line L1399 (-81.1546, -129.8648) -> (-78.6546, -129.8648)
  line L1400 (-60.9101, -131.2013) -> (-62.1601, -133.3664)
  line L1401 (-60.9101, -135.5315) -> (-58.4101, -135.5315)
  line L1402 (-73.6056, -126.9497) -> (-72.3556, -124.7847)
  line L1403 (-40.6657, -135.5315) -> (-38.1657, -135.5315)
  line L1404 (-47.0379, -133.3664) -> (-48.2879, -131.2013)
  line L1405 (-96.35, -122.6196) -> (-97.6, -124.7847)
  line L1406 (-41.9157, -133.3664) -> (-40.6657, -135.5315)
  line L1407 (-76.1056, -132.6164) -> (-73.6056, -132.6164)
  line L1408 (-73.6056, -128.2863) -> (-76.1056, -128.2863)
  line L1409 (-25.4944, -128.2863) -> (-26.7444, -130.4513)
  line L1410 (-58.4101, -135.5315) -> (-57.1601, -133.3664)
  line L1411 (-98.899, -125.5347) -> (-101.399, -125.5347)
  line L1412 (-71.0324, -135.5315) -> (-68.5324, -135.5315)
  line L1413 (-77.3556, -130.4513) -> (-76.1056, -132.6164)
  line L1414 (-52.0379, -133.3664) -> (-50.7879, -135.5315)
  line L1415 (-55.8611, -128.2863) -> (-57.1111, -130.4513)
  line L1416 (-65.9833, -132.6164) -> (-63.4833, -132.6164)
  line L1417 (-35.6167, -128.2863) -> (-36.8667, -130.4513)
  line L1418 (-78.6546, -125.5347) -> (-81.1546, -125.5347)
  line L1419 (-33.1167, -128.2863) -> (-35.6167, -128.2863)
  line L1420 (-36.8667, -130.4513) -> (-35.6167, -132.6164)
  line L1421 (-46.9889, -130.4513) -> (-45.7389, -132.6164)
  line L1422 (-5.25, -132.6164) -> (-2.75, -132.6164)
  line L1423 (-77.3556, -124.7847) -> (-76.1056, -126.9497)
  line L1424 (-35.6167, -132.6164) -> (-33.1167, -132.6164)
  line L1425 (-5.25, -128.2863) -> (-6.5, -130.4513)
  line L1426 (-31.7935, -133.3664) -> (-30.5435, -135.5315)
  line L1427 (-68.5324, -135.5315) -> (-67.2824, -133.3664)
  line L1428 (-68.5324, -131.2013) -> (-71.0324, -131.2013)
  line L1429 (-57.1111, -130.4513) -> (-55.8611, -132.6164)
  line L1430 (-31.8667, -130.4513) -> (-33.1167, -128.2863)
  line L1431 (-83.7278, -126.9497) -> (-82.4778, -124.7847)
  line L1432 (-28.0435, -131.2013) -> (-30.5435, -131.2013)
  line L1433 (-62.1601, -133.3664) -> (-60.9101, -135.5315)
  line L1434 (-57.1601, -133.3664) -> (-58.4101, -131.2013)
  line L1435 (-25.4944, -132.6164) -> (-22.9944, -132.6164)
  line L1436 (-77.4046, -133.3664) -> (-78.6546, -131.2013)
  line L1437 (-41.9889, -130.4513) -> (-43.2389, -128.2863)
  line L1438 (-21.6713, -139.0331) -> (-20.4213, -141.1981)
  line L1439 (-6.5, -136.118) -> (-5.25, -138.2831)
  line L1440 (-65.9833, -128.2863) -> (-67.2333, -130.4513)
  line L1441 (-87.4778, -130.4513) -> (-86.2278, -132.6164)
  line L1442 (-92.5268, -133.3664) -> (-91.2768, -135.5315)
  line L1443 (-7.799, -141.1981) -> (-6.549, -139.0331)
  line L1444 (-20.4213, -141.1981) -> (-17.9213, -141.1981)
  line L1445 (-25.4944, -133.9529) -> (-26.7444, -136.118)
  line L1446 (-76.1056, -128.2863) -> (-77.3556, -130.4513)
  line L1447 (-15.3722, -138.2831) -> (-12.8722, -138.2831)
  line L1448 (-17.9213, -141.1981) -> (-16.6713, -139.0331)
  line L1449 (-1.5, -136.118) -> (-2.75, -133.9529)
  line L1450 (-30.5435, -135.5315) -> (-28.0435, -135.5315)
  line L1451 (-6.549, -139.0331) -> (-7.799, -136.868)
  line L1452 (-30.5435, -136.868) -> (-31.7935, -139.0331)
  line L1453 (-101.399, -131.2013) -> (-102.649, -133.3664)
  line L1454 (-10.299, -136.868) -> (-11.549, -139.0331)
  line L1455 (-12.8722, -133.9529) -> (-15.3722, -133.9529)
  line L1456 (-72.2824, -133.3664) -> (-71.0324, -135.5315)
  line L1457 (-93.85, -132.6164) -> (-92.6, -130.4513)
  line L1458 (-21.7444, -130.4513) -> (-22.9944, -128.2863)
  line L1459 (-71.0324, -131.2013) -> (-72.2824, -133.3664)
  line L1460 (-40.6657, -131.2013) -> (-41.9157, -133.3664)
  line L1461 (-53.3611, -132.6164) -> (-52.1111, -130.4513)
  line L1462 (-48.2879, -131.2013) -> (-50.7879, -131.2013)
  line L1463 (-20.4213, -136.868) -> (-21.6713, -139.0331)
  line L1464 (-10.299, -141.1981) -> (-7.799, -141.1981)
  line L1465 (-21.7444, -136.118) -> (-22.9944, -133.9529)
  line L1466 (-5.25, -138.2831) -> (-2.75, -138.2831)
  line L1467 (-86.2278, -128.2863) -> (-87.4778, -130.4513)
  line L1468 (-86.2278, -132.6164) -> (-83.7278, -132.6164)
  line L1469 (-72.3556, -130.4513) -> (-73.6056, -128.2863)
  line L1470 (-16.6713, -139.0331) -> (-17.9213, -136.868)
  line L1471 (-28.0435, -135.5315) -> (-26.7935, -133.3664)
  line L1472 (-43.2389, -132.6164) -> (-41.9889, -130.4513)
  line L1473 (-33.1167, -132.6164) -> (-31.8667, -130.4513)
  line L1474 (-67.2333, -130.4513) -> (-65.9833, -132.6164)
  line L1475 (-93.85, -128.2863) -> (-96.35, -128.2863)
  line L1476 (-22.9944, -128.2863) -> (-25.4944, -128.2863)
  line L1477 (-22.9944, -133.9529) -> (-25.4944, -133.9529)
  line L1478 (-28.0435, -136.868) -> (-30.5435, -136.868)
  line L1479 (-26.7444, -136.118) -> (-25.4944, -138.2831)
  line L1480 (-31.7935, -139.0331) -> (-30.5435, -141.1981)
  line L1481 (-17.9213, -136.868) -> (-20.4213, -136.868)
  line L1482 (-38.1657, -131.2013) -> (-40.6657, -131.2013)
  line L1483 (-43.2389, -128.2863) -> (-45.7389, -128.2863)
  line L1484 (-98.899, -135.5315) -> (-97.649, -133.3664)
  line L1485 (-11.549, -139.0331) -> (-10.299, -141.1981)
  line L1486 (-81.1546, -135.5315) -> (-78.6546, -135.5315)
  line L1487 (-2.75, -133.9529) -> (-5.25, -133.9529)
  line L1488 (-25.4944, -138.2831) -> (-22.9944, -138.2831)
  line L1489 (-45.7389, -128.2863) -> (-46.9889, -130.4513)
  line L1490 (-92.6, -130.4513) -> (-93.85, -128.2863)
  line L1491 (-63.4833, -132.6164) -> (-62.2333, -130.4513)
  line L1492 (-52.1111, -130.4513) -> (-53.3611, -128.2863)
  line L1493 (-53.3611, -128.2863) -> (-55.8611, -128.2863)
  line L1494 (-16.6222, -136.118) -> (-15.3722, -138.2831)
  line L1495 (-58.4101, -131.2013) -> (-60.9101, -131.2013)
  line L1496 (-88.7768, -131.2013) -> (-91.2768, -131.2013)
  line L1497 (-78.6546, -135.5315) -> (-77.4046, -133.3664)
  line L1498 (-11.6222, -136.118) -> (-12.8722, -133.9529)
  line L1499 (-22.9944, -138.2831) -> (-21.7444, -136.118)
  line L1500 (-2.75, -138.2831) -> (-1.5, -136.118)
  line L1501 (-28.0435, -141.1981) -> (-26.7935, -139.0331)
  line L1502 (-96.35, -132.6164) -> (-93.85, -132.6164)
  line L1503 (-36.8667, -136.118) -> (-35.6167, -138.2831)
  line L1504 (-33.1167, -133.9529) -> (-35.6167, -133.9529)
  line L1505 (-12.8722, -138.2831) -> (-11.6222, -136.118)
  line L1506 (-71.0324, -141.1981) -> (-68.5324, -141.1981)
  line L1507 (-78.6546, -136.868) -> (-81.1546, -136.868)
  line L1508 (-40.6657, -141.1981) -> (-38.1657, -141.1981)
  line L1509 (-81.1546, -136.868) -> (-82.4046, -139.0331)
  line L1510 (-15.3722, -133.9529) -> (-16.6222, -136.118)
  line L1511 (-102.649, -133.3664) -> (-101.399, -135.5315)
  line L1512 (-87.5268, -133.3664) -> (-88.7768, -131.2013)
  line L1513 (-52.1111, -136.118) -> (-53.3611, -133.9529)
  line L1514 (-71.0324, -136.868) -> (-72.2824, -139.0331)
  line L1515 (-98.899, -131.2013) -> (-101.399, -131.2013)
  line L1516 (-45.7389, -138.2831) -> (-43.2389, -138.2831)
  line L1517 (-91.2768, -135.5315) -> (-88.7768, -135.5315)
  line L1518 (-38.1657, -136.868) -> (-40.6657, -136.868)
  line L1519 (-58.4101, -141.1981) -> (-57.1601, -139.0331)
  line L1520 (-96.35, -128.2863) -> (-97.6, -130.4513)
  line L1521 (-47.0379, -139.0331) -> (-48.2879, -136.868)
  line L1522 (-30.5435, -141.1981) -> (-28.0435, -141.1981)
  line L1523 (-41.9157, -139.0331) -> (-40.6657, -141.1981)
  line L1524 (-83.7278, -132.6164) -> (-82.4778, -130.4513)
  line L1525 (-46.9889, -136.118) -> (-45.7389, -138.2831)
  line L1526 (-55.8611, -133.9529) -> (-57.1111, -136.118)
  line L1527 (-97.649, -133.3664) -> (-98.899, -131.2013)
  line L1528 (-63.4833, -138.2831) -> (-62.2333, -136.118)
  line L1529 (-77.3556, -136.118) -> (-76.1056, -138.2831)
  line L1530 (-78.6546, -131.2013) -> (-81.1546, -131.2013)
  line L1531 (-38.1657, -141.1981) -> (-36.9157, -139.0331)
  line L1532 (-43.2389, -138.2831) -> (-41.9889, -136.118)
  line L1533 (-82.4046, -133.3664) -> (-81.1546, -135.5315)
  line L1534 (-62.1601, -139.0331) -> (-60.9101, -141.1981)
  line L1535 (-57.1601, -139.0331) -> (-58.4101, -136.868)
  line L1536 (-45.7389, -133.9529) -> (-46.9889, -136.118)
  line L1537 (-50.7879, -136.868) -> (-52.0379, -139.0331)
  line L1538 (-58.4101, -136.868) -> (-60.9101, -136.868)
  line L1539 (-91.2768, -131.2013) -> (-92.5268, -133.3664)
  line L1540 (-48.2879, -141.1981) -> (-47.0379, -139.0331)
  line L1541 (-68.5324, -141.1981) -> (-67.2824, -139.0331)
  line L1542 (-43.2389, -133.9529) -> (-45.7389, -133.9529)
  line L1543 (-53.3611, -138.2831) -> (-52.1111, -136.118)
  line L1544 (-82.4046, -139.0331) -> (-81.1546, -141.1981)
  line L1545 (-36.9157, -139.0331) -> (-38.1657, -136.868)
  line L1546 (-7.799, -136.868) -> (-10.299, -136.868)
  line L1547 (-55.8611, -138.2831) -> (-53.3611, -138.2831)
  line L1548 (-97.6, -130.4513) -> (-96.35, -132.6164)
  line L1549 (-65.9833, -138.2831) -> (-63.4833, -138.2831)
  line L1550 (-101.399, -135.5315) -> (-98.899, -135.5315)
  line L1551 (-41.9889, -136.118) -> (-43.2389, -133.9529)
  line L1552 (-72.3556, -136.118) -> (-73.6056, -133.9529)
  line L1553 (-83.7278, -128.2863) -> (-86.2278, -128.2863)
  line L1554 (-67.2824, -139.0331) -> (-68.5324, -136.868)
  line L1555 (-73.6056, -138.2831) -> (-72.3556, -136.118)
  line L1556 (-81.1546, -131.2013) -> (-82.4046, -133.3664)
  line L1557 (-88.7768, -135.5315) -> (-87.5268, -133.3664)
  line L1558 (-35.6167, -138.2831) -> (-33.1167, -138.2831)
  line L1559 (-62.2333, -136.118) -> (-63.4833, -133.9529)
  line L1560 (-82.4778, -130.4513) -> (-83.7278, -128.2863)
  line L1561 (-76.1056, -133.9529) -> (-77.3556, -136.118)
  line L1562 (-52.0379, -139.0331) -> (-50.7879, -141.1981)
  line L1563 (-5.25, -133.9529) -> (-6.5, -136.118)
  line L1564 (-26.7935, -144.6997) -> (-28.0435, -142.5347)
  line L1565 (-28.0435, -142.5347) -> (-30.5435, -142.5347)
  line L1566 (-20.4213, -142.5347) -> (-21.6713, -144.6997)
  line L1567 (-12.8722, -143.9497) -> (-11.6222, -141.7847)
  line L1568 (-25.4944, -139.6196) -> (-26.7444, -141.7847)
  line L1569 (-91.2768, -136.868) -> (-92.5268, -139.0331)
  line L1570 (-35.6167, -139.6196) -> (-36.8667, -141.7847)
  line L1571 (-60.9101, -136.868) -> (-62.1601, -139.0331)
  line L1572 (-30.5435, -142.5347) -> (-31.7935, -144.6997)
  line L1573 (-31.8667, -136.118) -> (-33.1167, -133.9529)
  line L1574 (-73.6056, -133.9529) -> (-76.1056, -133.9529)
  line L1575 (-33.1167, -138.2831) -> (-31.8667, -136.118)
  line L1576 (-6.5, -141.7847) -> (-5.25, -143.9497)
  line L1577 (-30.5435, -146.8648) -> (-28.0435, -146.8648)
  line L1578 (-10.299, -142.5347) -> (-11.549, -144.6997)